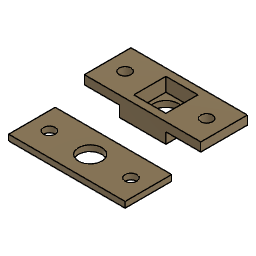
Soporte_Poten v4 (Autodesk Fusion 360 design; units mm, degrees)
Autodesk Fusion 360 part; units mm, degrees
note: some values were not read from the file. Set by a fixed rule: which sketch regions a step uses.
sketch "Boceto1" plane through (0, 0, 0) normal (0, 0, 1) x (1, 0, 0)
  circle A0 centre (0, 0) radius 4.25
  line L0 (8, 8) -> (-8, 8)
  line L1 (-8, 8) -> (-8, -8)
  line L2 (-8, -8) -> (8, -8)
  line L3 (8, -8) -> (8, 8)
  line L4 (8, 8) -> (-8, -8) construction
  line L5 (-8, 8) -> (8, -8) construction
  dimension "d1" = 8.5
  dimension "d39" = 16
  dimension "d40" = 16
  constraint coincident A0.centre origin
  constraint horizontal L0
  constraint perpendicular L0 L1
  constraint parallel L0 L2
  constraint parallel L1 L3
  constraint coincident L4 A0.centre
  constraint coincident L5 A0.centre
  measures "d1" diameter of A0
  measures "d39" distance of L1.end L2.end
  measures "d40" distance of L0.end L1.end
extrude "Extruir1" add sketch "Boceto1" along normal blind 2 makes body 1
sketch "Boceto2" plane through (0, 0, 2) normal (0, 0, 1) x (-1, 0, 0)
  line L0 (8, -8) -> (-8, -8)
  line L1 (-8, -8) -> (-8, 8)
  line L2 (-8, 8) -> (8, 8)
  line L3 (8, 8) -> (8, -8)
  line L4 (8, -8) -> (-8, 8) construction
  line L5 (-8, -8) -> (8, 8) construction
  line L6 (5.5, 5.5) -> (5.5, -5.5)
  line L7 (5.5, -5.5) -> (-5.5, -5.5)
  line L8 (-5.5, -5.5) -> (-5.5, 5.5)
  line L9 (-5.5, 5.5) -> (5.5, 5.5)
  dimension "d24" = 16
  dimension "d25" = 2.5
  dimension "d26" = 8
  constraint horizontal L0
  constraint perpendicular L0 L1
  constraint parallel L0 L2
  constraint parallel L1 L3
  constraint coincident L4 origin
  constraint coincident L5 origin
  measures "d24" distance of L1.end L2.end
  measures "d26" distance of L0 origin
extrude "Extruir2" add sketch "Boceto2" along normal blind 1.7 bodies 1
sketch "Boceto3" plane through (0, 0, 3.7) normal (0, 0, 1) x (-1, 0, 0)
  line L0 (-20, -8) -> (20, -8)
  line L1 (20, -8) -> (20, 8)
  line L2 (20, 8) -> (-20, 8)
  line L3 (-20, 8) -> (-20, -8)
  line L4 (-20, -8) -> (20, 8) construction
  line L5 (20, -8) -> (-20, 8) construction
  circle A0 centre (-14, 0) radius 2
  circle A1 centre (14, 0) radius 2
  line L6 (-5.5, -5.5) -> (-5.5, 5.5)
  line L7 (-5.5, 5.5) -> (5.5, 5.5)
  line L8 (5.5, 5.5) -> (5.5, -5.5)
  line L9 (5.5, -5.5) -> (-5.5, -5.5)
  line L10 (8, 8) -> (-8, 8)
  line L11 (-8, 8) -> (-8, -8)
  line L12 (-8, -8) -> (8, -8)
  line L13 (8, -8) -> (8, 8)
  dimension "d16" = 40
  dimension "d17" = 16
  dimension "d18" = 4
  dimension "d19" = 4
  dimension "d20" = 14
  dimension "d21" = 14
  constraint horizontal L0
  constraint perpendicular L0 L1
  constraint parallel L0 L2
  constraint parallel L1 L3
  constraint coincident L4 origin
  constraint coincident L5 origin
  constraint horizontal A0.centre A1.centre
  constraint collinear origin A0.centre A1.centre
  measures "d16" distance of L1.end L2.end
  measures "d17" distance of L0.end L1.end
  measures "d18" diameter of A0
  measures "d19" diameter of A1
  measures "d20" distance of origin A0.centre
  measures "d21" distance of origin A1.centre
extrude "Extruir3" add sketch "Boceto3" along normal blind 3 bodies 1
sketch "Boceto5" plane through (0, 0, 0) normal (0, 0, 1) x (1, 0, 0)
  line L0 (20, -18) -> (-20, -18)
  line L1 (-20, -18) -> (-20, -34)
  line L2 (-20, -34) -> (20, -34)
  line L3 (20, -34) -> (20, -18)
  line L4 (20, -18) -> (-20, -34) construction
  line L5 (-20, -18) -> (20, -34) construction
  line L6 (-20, -8) -> (20, -8)
  circle A0 centre (14, -26) radius 2
  circle A1 centre (-14, -26) radius 2
  circle A2 centre (0, -26) radius 4
  point P0 (0, -26)
  dimension "d27" = 40
  dimension "d28" = 16
  dimension "d29" = 10
  dimension "d30" = 4
  dimension "d31" = 4
  dimension "d32" = 14
  dimension "d33" = 14
  dimension "d34" = 8
  dimension "d35" = 26
  dimension "d36" = 26
  constraint horizontal L0
  constraint perpendicular L0 L1
  constraint parallel L0 L2
  constraint parallel L1 L3
  constraint coincident L4 P0
  constraint coincident L5 P0
  constraint coincident P0 A2.centre
  constraint collinear P0 A0.centre A1.centre
  measures "d27" distance of L1.end L2.end
  measures "d28" distance of L0.end L1.end
  measures "d29" distance of L0 L6
  measures "d30" diameter of A0
  measures "d31" diameter of A1
  measures "d32" distance of P0 A0.centre
  measures "d33" distance of P0 A1.centre
  measures "d34" diameter of A2
  measures "d35" distance of origin A2.centre
  measures "d36" vertical distance of origin A0.centre
extrude "Extruir4" add sketch "Boceto5" along normal blind 2 separate body makes body 2
